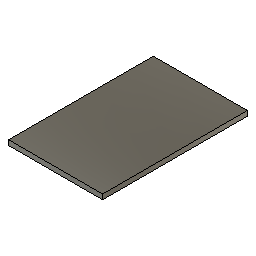
Bottom Standing Plate v2 (Autodesk Fusion 360 design; units mm, degrees)
Autodesk Fusion 360 part; units mm, degrees
sketch "Sketch1" plane through (0, 0, 0) normal (0, 0, 1) x (1, 0, 0)
  line L0 (0, 0) -> (358.775, 0)
  line L1 (358.775, 0) -> (358.775, -552.45)
  line L2 (358.775, -552.45) -> (0, -552.45)
  line L3 (0, -552.45) -> (0, 0)
  dimension "d3" = 552.45
  dimension "d4" = 358.775
  constraint horizontal L0
  constraint vertical L1
  constraint horizontal L2
  constraint vertical L3
  constraint coincident L0.start L3.end
  measures "d3" distance of L0.start L2.end
  measures "d4" distance of L0.start L0.end
extrude "Extrude1" add sketch "Sketch1" along normal blind 19.05
